Autodesk Inventor part; units mm, degrees
(part 2 of 2)
  line L680 (-7.1521, 71.8798) -> (-10.036, 76.875)
  line L681 (-4.554, 73.3798) -> (-7.4379, 78.375)
  line L682 (4.0979, 78.375) -> (1.214, 83.3701)
  line L683 (1.214, 83.3701) -> (-1.67, 83.3701)
  line L684 (-4.554, 83.3701) -> (-1.67, 83.3701)
  line L685 (-10.036, 76.875) -> (-15.804, 76.875)
  line L686 (-10.036, 79.875) -> (-15.804, 79.875)
  line L687 (-7.4379, 78.375) -> (-4.554, 83.3701)
  line L688 (-7.1521, 84.8701) -> (-10.036, 79.875)
  line L689 (3.8121, 84.8701) -> (6.696, 79.875)
  line L690 (60.0621, 65.3846) -> (62.946, 70.3798)
  line L691 (57.464, 66.8846) -> (60.3479, 71.8798)
  line L692 (62.946, 60.3894) -> (60.0621, 65.3846)
  line L693 (57.464, 63.8846) -> (60.3479, 58.8894)
  line L694 (51.696, 63.8846) -> (57.464, 63.8846)
  line L695 (51.696, 66.8846) -> (57.464, 66.8846)
  line L696 (51.696, 76.875) -> (57.464, 76.875)
  line L697 (51.696, 79.875) -> (57.464, 79.875)
  line L698 (57.464, 76.875) -> (60.3479, 71.8798)
  line L699 (60.0621, 78.375) -> (62.946, 73.3798)
  line L700 (62.946, 83.3701) -> (60.0621, 78.375)
  line L701 (57.464, 79.875) -> (60.3479, 84.8701)
  line L702 (23.714, 73.3798) -> (20.83, 73.3798)
  line L703 (29.196, 76.875) -> (26.3121, 71.8798)
  line L704 (26.5979, 78.375) -> (23.714, 73.3798)
  line L705 (34.964, 76.875) -> (29.196, 76.875)
  line L706 (20.83, 83.3701) -> (23.714, 83.3701)
  line L707 (23.714, 83.3701) -> (26.5979, 78.375)
  line L708 (34.964, 79.875) -> (29.196, 79.875)
  line L709 (29.196, 79.875) -> (26.3121, 84.8701)
  line L710 (37.8479, 84.8701) -> (34.964, 79.875)
  line L711 (37.8479, 71.8798) -> (34.964, 76.875)
  line L712 (6.696, 63.8846) -> (12.464, 63.8846)
  line L713 (6.696, 66.8846) -> (12.464, 66.8846)
  line L714 (6.696, 76.875) -> (12.464, 76.875)
  line L715 (6.696, 79.875) -> (12.464, 79.875)
  line L716 (12.464, 79.875) -> (15.3479, 84.8701)
  line L717 (12.464, 76.875) -> (15.3479, 71.8798)
  line L718 (17.946, 83.3701) -> (15.0621, 78.375)
  line L719 (20.83, 83.3701) -> (17.946, 83.3701)
  line L720 (15.0621, 78.375) -> (17.946, 73.3798)
  line L721 (17.946, 73.3798) -> (20.83, 73.3798)
  line L722 (-29.9379, 78.375) -> (-27.054, 83.3701)
  line L723 (-33.4021, 78.375) -> (-29.6521, 84.8701)
  line L724 (-27.054, 83.3701) -> (-21.286, 83.3701)
  line L725 (-21.286, 83.3701) -> (-18.4021, 78.375)
  line L726 (-15.804, 79.875) -> (-18.6879, 84.8701)
  line L727 (48.8121, 71.8798) -> (51.696, 76.875)
  line L728 (43.33, 73.3798) -> (40.446, 73.3798)
  line L729 (46.214, 73.3798) -> (49.0979, 78.375)
  line L730 (40.446, 73.3798) -> (37.5621, 78.375)
  line L731 (43.33, 73.3798) -> (46.214, 73.3798)
  line L732 (51.696, 11.923) -> (57.464, 11.923)
  line L733 (62.946, 8.4279) -> (60.0621, 13.423)
  line L734 (57.464, 11.923) -> (60.3479, 6.9279)
  line L735 (4.0979, 52.3942) -> (1.214, 57.3894)
  line L736 (-1.67, 47.399) -> (1.214, 47.399)
  line L737 (1.214, 57.3894) -> (-1.67, 57.3894)
  line L738 (-1.67, 47.399) -> (-4.554, 47.399)
  line L739 (-4.554, 57.3894) -> (-1.67, 57.3894)
  line L740 (-4.554, 47.399) -> (-7.4379, 52.3942)
  line L741 (-7.1521, 45.899) -> (-10.036, 50.8942)
  line L742 (-7.4379, 52.3942) -> (-4.554, 57.3894)
  line L743 (-7.1521, 58.8894) -> (-10.036, 53.8942)
  line L744 (1.214, 47.399) -> (4.0979, 52.3942)
  line L745 (-7.1521, 19.9182) -> (-10.036, 14.923)
  line L746 (-7.1521, 6.9279) -> (-10.036, 11.923)
  line L747 (-1.67, 18.4182) -> (-4.554, 18.4182)
  line L748 (-1.67, 18.4182) -> (1.214, 18.4182)
  line L749 (-4.554, 18.4182) -> (-7.4379, 13.423)
  line L750 (-7.4379, 13.423) -> (-4.554, 8.4279)
  line L751 (-4.554, 8.4279) -> (-1.67, 8.4279)
  line L752 (1.214, 8.4279) -> (-1.67, 8.4279)
  line L753 (4.0979, 13.423) -> (1.214, 8.4279)
  line L754 (3.8121, 6.9279) -> (6.696, 11.923)
  line L755 (26.5979, 13.423) -> (23.714, 18.4182)
  line L756 (23.714, 8.4279) -> (26.5979, 13.423)
  line L757 (20.83, 8.4279) -> (23.714, 8.4279)
  line L758 (23.714, 18.4182) -> (20.83, 18.4182)
  line L759 (20.83, 8.4279) -> (17.946, 8.4279)
  line L760 (17.946, 18.4182) -> (20.83, 18.4182)
  line L761 (17.946, 8.4279) -> (15.0621, 13.423)
  line L762 (12.464, 11.923) -> (15.3479, 6.9279)
  line L763 (15.0621, 13.423) -> (17.946, 18.4182)
  line L764 (12.464, 14.923) -> (15.3479, 19.9182)
  line L765 (29.196, 14.923) -> (26.3121, 19.9182)
  line L766 (29.196, 11.923) -> (26.3121, 6.9279)
  line L767 (34.964, 14.923) -> (29.196, 14.923)
  line L768 (34.964, 11.923) -> (29.196, 11.923)
  line L769 (43.33, 21.4182) -> (40.446, 21.4182)
  line L770 (43.33, 21.4182) -> (46.214, 21.4182)
  line L771 (43.33, 18.4182) -> (40.446, 18.4182)
  line L772 (43.33, 18.4182) -> (46.214, 18.4182)
  line L773 (37.8479, 19.9182) -> (34.964, 14.923)
  line L774 (40.446, 18.4182) -> (37.5621, 13.423)
  line L775 (48.8121, 19.9182) -> (51.696, 14.923)
  line L776 (46.214, 18.4182) -> (49.0979, 13.423)
  line L777 (37.8479, 6.9279) -> (34.964, 11.923)
  line L778 (37.5621, 13.423) -> (40.446, 8.4279)
  line L779 (40.446, 8.4279) -> (43.33, 8.4279)
  line L780 (46.214, 8.4279) -> (43.33, 8.4279)
  line L781 (49.0979, 13.423) -> (46.214, 8.4279)
  line L782 (48.8121, 6.9279) -> (51.696, 11.923)
  line L783 (-18.4021, 26.4134) -> (-21.286, 21.4182)
  line L784 (-15.804, 24.9134) -> (-18.6879, 19.9182)
  line L785 (-18.4021, 13.423) -> (-21.286, 18.4182)
  line L786 (-21.286, 8.4279) -> (-18.4021, 13.423)
  line L787 (-15.804, 11.923) -> (-18.6879, 6.9279)
  line L788 (-10.036, 11.923) -> (-15.804, 11.923)
  line L789 (-10.036, 14.923) -> (-15.804, 14.923)
  line L790 (-15.804, 14.923) -> (-18.6879, 19.9182)
  line L791 (-27.054, 8.4279) -> (-21.286, 8.4279)
  line L792 (-21.286, 21.4182) -> (-27.054, 21.4182)
  line L793 (-21.286, 18.4182) -> (-27.054, 18.4182)
  line L794 (-29.9379, 13.423) -> (-27.054, 8.4279)
  line L795 (-27.054, 18.4182) -> (-29.9379, 13.423)
  line L796 (-27.054, 21.4182) -> (-29.9379, 26.4134)
  line L797 (-32.969, 14.173) -> (-29.6521, 19.9182)
  line L798 (-29.6521, 19.9182) -> (-33.4021, 26.4134)
  line L799 (46.214, 21.4182) -> (49.0979, 26.4134)
  line L800 (37.8479, 19.9182) -> (34.964, 24.9134)
  line L801 (40.446, 21.4182) -> (37.5621, 26.4134)
  line L802 (37.5621, 26.4134) -> (40.446, 31.4086)
  line L803 (37.8479, 32.9086) -> (34.964, 27.9134)
  line L804 (-1.67, 21.4182) -> (1.214, 21.4182)
  line L805 (-1.67, 21.4182) -> (-4.554, 21.4182)
  line L806 (-7.1521, 19.9182) -> (-10.036, 24.9134)
  line L807 (-4.554, 21.4182) -> (-7.4379, 26.4134)
  line L808 (1.214, 31.4086) -> (-1.67, 31.4086)
  line L809 (-7.4379, 26.4134) -> (-4.554, 31.4086)
  line L810 (-7.1521, 32.9086) -> (-10.036, 27.9134)
  line L811 (23.714, 21.4182) -> (20.83, 21.4182)
  line L812 (17.946, 21.4182) -> (20.83, 21.4182)
  line L813 (29.196, 24.9134) -> (26.3121, 19.9182)
  line L814 (12.464, 24.9134) -> (15.3479, 19.9182)
  line L815 (15.0621, 26.4134) -> (17.946, 21.4182)
  line L816 (26.5979, 26.4134) -> (23.714, 21.4182)
  line L817 (34.964, 24.9134) -> (29.196, 24.9134)
  line L818 (34.964, 27.9134) -> (29.196, 27.9134)
  line L819 (20.83, 31.4086) -> (23.714, 31.4086)
  line L820 (23.714, 31.4086) -> (26.5979, 26.4134)
  line L821 (29.196, 27.9134) -> (26.3121, 32.9086)
  line L822 (1.214, 18.4182) -> (4.0979, 13.423)
  line L823 (3.8121, 19.9182) -> (6.696, 14.923)
  line L824 (6.696, 11.923) -> (12.464, 11.923)
  line L825 (6.696, 14.923) -> (12.464, 14.923)
  line L826 (1.214, 21.4182) -> (4.0979, 26.4134)
  line L827 (3.8121, 19.9182) -> (6.696, 24.9134)
  line L828 (4.0979, 26.4134) -> (1.214, 31.4086)
  line L829 (3.8121, 32.9086) -> (6.696, 27.9134)
  line L830 (6.696, 24.9134) -> (12.464, 24.9134)
  line L831 (6.696, 27.9134) -> (12.464, 27.9134)
  line L832 (12.464, 27.9134) -> (15.3479, 32.9086)
  line L833 (17.946, 31.4086) -> (15.0621, 26.4134)
  line L834 (57.464, 37.9038) -> (60.3479, 32.9086)
  line L835 (62.946, 34.4086) -> (60.0621, 39.4038)
  line L836 (51.696, 37.9038) -> (57.464, 37.9038)
  line L837 (51.696, 40.9038) -> (57.464, 40.9038)
  line L838 (60.0621, 39.4038) -> (62.946, 44.399)
  line L839 (57.464, 40.9038) -> (60.3479, 45.899)
  line L840 (46.214, 31.4086) -> (43.33, 31.4086)
  line L841 (40.446, 31.4086) -> (43.33, 31.4086)
  line L842 (48.8121, 32.9086) -> (51.696, 37.9038)
  line L843 (46.214, 34.4086) -> (43.33, 34.4086)
  line L844 (49.0979, 39.4038) -> (46.214, 34.4086)
  line L845 (40.446, 34.4086) -> (43.33, 34.4086)
  line L846 (48.8121, 45.899) -> (51.696, 40.9038)
  line L847 (46.214, 44.399) -> (49.0979, 39.4038)
  line L848 (43.33, 44.399) -> (46.214, 44.399)
  line L849 (43.33, 44.399) -> (40.446, 44.399)
  line L850 (20.83, 34.4086) -> (23.714, 34.4086)
  line L851 (29.196, 37.9038) -> (26.3121, 32.9086)
  line L852 (34.964, 37.9038) -> (29.196, 37.9038)
  line L853 (37.8479, 32.9086) -> (34.964, 37.9038)
  line L854 (23.714, 34.4086) -> (26.5979, 39.4038)
  line L855 (34.964, 40.9038) -> (29.196, 40.9038)
  line L856 (37.5621, 39.4038) -> (40.446, 34.4086)
  line L857 (23.714, 44.399) -> (20.83, 44.399)
  line L858 (26.5979, 39.4038) -> (23.714, 44.399)
  line L859 (29.196, 40.9038) -> (26.3121, 45.899)
  line L860 (40.446, 44.399) -> (37.5621, 39.4038)
  line L861 (37.8479, 45.899) -> (34.964, 40.9038)
  line L862 (3.8121, 45.899) -> (6.696, 40.9038)
  line L863 (1.214, 44.399) -> (4.0979, 39.4038)
  line L864 (6.696, 40.9038) -> (12.464, 40.9038)
  line L865 (6.696, 37.9038) -> (12.464, 37.9038)
  line L866 (4.0979, 39.4038) -> (1.214, 34.4086)
  line L867 (3.8121, 32.9086) -> (6.696, 37.9038)
  line L868 (-15.804, 27.9134) -> (-18.6879, 32.9086)
  line L869 (-10.036, 27.9134) -> (-15.804, 27.9134)
  line L870 (-10.036, 24.9134) -> (-15.804, 24.9134)
  line L871 (-4.554, 31.4086) -> (-1.67, 31.4086)
  line L872 (-15.804, 40.9038) -> (-18.6879, 45.899)
  line L873 (-10.036, 40.9038) -> (-15.804, 40.9038)
  line L874 (-15.804, 37.9038) -> (-18.6879, 32.9086)
  line L875 (-10.036, 37.9038) -> (-15.804, 37.9038)
  line L876 (-7.1521, 45.899) -> (-10.036, 40.9038)
  line L877 (-1.67, 44.399) -> (-4.554, 44.399)
  line L878 (-4.554, 44.399) -> (-7.4379, 39.4038)
  line L879 (-7.1521, 32.9086) -> (-10.036, 37.9038)
  line L880 (-1.67, 44.399) -> (1.214, 44.399)
  line L881 (-7.4379, 39.4038) -> (-4.554, 34.4086)
  line L882 (-4.554, 34.4086) -> (-1.67, 34.4086)
  line L883 (1.214, 34.4086) -> (-1.67, 34.4086)
  line L884 (20.83, 31.4086) -> (17.946, 31.4086)
  line L885 (12.464, 37.9038) -> (15.3479, 32.9086)
  line L886 (20.83, 34.4086) -> (17.946, 34.4086)
  line L887 (17.946, 34.4086) -> (15.0621, 39.4038)
  line L888 (15.0621, 39.4038) -> (17.946, 44.399)
  line L889 (17.946, 44.399) -> (20.83, 44.399)
  line L890 (17.946, 47.399) -> (20.83, 47.399)
  line L891 (12.464, 40.9038) -> (15.3479, 45.899)
  line L892 (48.8121, 45.899) -> (51.696, 50.8942)
  line L893 (51.696, 50.8942) -> (57.464, 50.8942)
  line L894 (51.696, 53.8942) -> (57.464, 53.8942)
  line L895 (57.464, 50.8942) -> (60.3479, 45.899)
  line L896 (60.0621, 52.3942) -> (62.946, 47.399)
  line L897 (62.946, 57.3894) -> (60.0621, 52.3942)
  line L898 (57.464, 53.8942) -> (60.3479, 58.8894)
  line L899 (48.8121, 58.8894) -> (51.696, 53.8942)
  line L900 (29.196, 53.8942) -> (26.3121, 58.8894)
  line L901 (29.196, 50.8942) -> (26.3121, 45.899)
  line L902 (34.964, 50.8942) -> (29.196, 50.8942)
  line L903 (34.964, 53.8942) -> (29.196, 53.8942)
  line L904 (37.8479, 45.899) -> (34.964, 50.8942)
  line L905 (37.8479, 58.8894) -> (34.964, 53.8942)
  line L906 (49.0979, 52.3942) -> (46.214, 57.3894)
  line L907 (46.214, 47.399) -> (49.0979, 52.3942)
  line L908 (46.214, 57.3894) -> (43.33, 57.3894)
  line L909 (40.446, 57.3894) -> (43.33, 57.3894)
  line L910 (43.33, 47.399) -> (40.446, 47.399)
  line L911 (37.5621, 52.3942) -> (40.446, 57.3894)
  line L912 (40.446, 47.399) -> (37.5621, 52.3942)
  line L913 (43.33, 47.399) -> (46.214, 47.399)
  line L914 (20.83, 57.3894) -> (17.946, 57.3894)
  line L915 (20.83, 57.3894) -> (23.714, 57.3894)
  line L916 (23.714, 57.3894) -> (26.5979, 52.3942)
  line L917 (12.464, 53.8942) -> (15.3479, 58.8894)
  line L918 (17.946, 57.3894) -> (15.0621, 52.3942)
  line L919 (6.696, 53.8942) -> (12.464, 53.8942)
  line L920 (3.8121, 58.8894) -> (6.696, 53.8942)
  line L921 (26.5979, 52.3942) -> (23.714, 47.399)
  line L922 (23.714, 47.399) -> (20.83, 47.399)
  line L923 (6.696, 50.8942) -> (12.464, 50.8942)
  line L924 (15.0621, 52.3942) -> (17.946, 47.399)
  line L925 (12.464, 50.8942) -> (15.3479, 45.899)
  line L926 (3.8121, 45.899) -> (6.696, 50.8942)
  line L927 (-18.4021, 52.3942) -> (-21.286, 47.399)
  line L928 (-32.969, 51.6442) -> (-29.6521, 45.899)
  line L929 (-27.054, 47.399) -> (-29.9379, 52.3942)
  line L930 (-21.286, 47.399) -> (-27.054, 47.399)
  line L931 (-15.804, 50.8942) -> (-18.6879, 45.899)
  line L932 (-10.036, 50.8942) -> (-15.804, 50.8942)
  line L933 (-10.036, 53.8942) -> (-15.804, 53.8942)
  line L934 (-21.286, 57.3894) -> (-18.4021, 52.3942)
  line L935 (-27.054, 57.3894) -> (-21.286, 57.3894)
  line L936 (-29.9379, 52.3942) -> (-27.054, 57.3894)
  line L937 (-15.804, 53.8942) -> (-18.6879, 58.8894)
  line L938 (49.0979, 26.4134) -> (46.214, 31.4086)
  line L939 (48.8121, 32.9086) -> (51.696, 27.9134)
  line L940 (51.696, 27.9134) -> (57.464, 27.9134)
  line L941 (48.8121, 19.9182) -> (51.696, 24.9134)
  line L942 (57.464, 27.9134) -> (60.3479, 32.9086)
  line L943 (51.696, 24.9134) -> (57.464, 24.9134)
  line L944 (62.946, 31.4086) -> (60.0621, 26.4134)
  line L945 (57.464, 24.9134) -> (60.3479, 19.9182)
  line L946 (51.696, 14.923) -> (57.464, 14.923)
  line L947 (57.464, 14.923) -> (60.3479, 19.9182)
  line L948 (60.0621, 13.423) -> (62.946, 18.4182)
  line L949 (60.0621, 26.4134) -> (62.946, 21.4182)
  line L950 (-21.286, 31.4086) -> (-18.4021, 26.4134)
  line L951 (-29.9379, 26.4134) -> (-27.054, 31.4086)
  line L952 (-33.4021, 26.4134) -> (-29.6521, 32.9086)
  line L953 (-27.054, 31.4086) -> (-21.286, 31.4086)
  line L954 (-27.054, 34.4086) -> (-21.286, 34.4086)
  line L955 (-33.4021, 39.4038) -> (-29.6521, 32.9086)
  line L956 (-29.9379, 39.4038) -> (-27.054, 34.4086)
  line L957 (-21.286, 34.4086) -> (-18.4021, 39.4038)
  line L958 (-18.4021, 39.4038) -> (-21.286, 44.399)
  line L959 (-21.286, 44.399) -> (-27.054, 44.399)
  line L960 (-27.054, 44.399) -> (-29.9379, 39.4038)
  line L961 (-29.6521, 45.899) -> (-33.4021, 39.4038)
  line L962 (-32.969, -39.2885) -> (-29.6521, -45.0337)
  line L963 (-29.6521, -45.0337) -> (-32.969, -50.7789)
  line L964 (-29.6521, 6.9279) -> (-32.969, 1.1827)
  line L965 (-29.6521, 6.9279) -> (-32.969, 12.673)
  line L966 (-32.969, 64.6346) -> (-29.6521, 58.8894)
  line L967 (-29.6521, 58.8894) -> (-32.969, 53.1442)
  line L968 (-32.969, 64.6346) -> (-33.4021, 65.3846)
  line L969 (-32.969, 66.1346) -> (-33.4021, 65.3846)
  line L970 (-32.969, 51.6442) -> (-33.4021, 52.3942)
  line L971 (-32.969, 53.1442) -> (-33.4021, 52.3942)
  line L972 (37.8479, 136.8317) -> (34.964, 141.8269)
  line L973 (37.5621, 143.3269) -> (40.446, 138.3317)
  line L974 (40.446, 138.3317) -> (43.33, 138.3317)
  line L975 (46.214, 138.3317) -> (43.33, 138.3317)
  line L976 (20.83, 135.3317) -> (17.946, 135.3317)
  line L977 (17.946, 138.3317) -> (15.0621, 143.3269)
  line L978 (20.83, 138.3317) -> (17.946, 138.3317)
  line L979 (20.83, 138.3317) -> (23.714, 138.3317)
  line L980 (23.714, 138.3317) -> (26.5979, 143.3269)
  line L981 (29.196, 141.8269) -> (26.3121, 136.8317)
  line L982 (6.696, 128.8365) -> (12.464, 128.8365)
  line L983 (6.696, 131.8365) -> (12.464, 131.8365)
  line L984 (17.946, 135.3317) -> (15.0621, 130.3365)
  line L985 (12.464, 131.8365) -> (15.3479, 136.8317)
  line L986 (6.696, 141.8269) -> (12.464, 141.8269)
  line L987 (12.464, 141.8269) -> (15.3479, 136.8317)
  line L988 (3.8121, 136.8317) -> (6.696, 141.8269)
  line L989 (4.0979, 143.3269) -> (1.214, 138.3317)
  line L990 (34.964, 141.8269) -> (29.196, 141.8269)
  line L991 (-7.4379, 117.3461) -> (-4.554, 112.3509)
  line L992 (-10.036, 118.8461) -> (-15.804, 118.8461)
  line L993 (-10.036, 115.8461) -> (-15.804, 115.8461)
  line L994 (-15.804, 115.8461) -> (-18.6879, 110.8509)
  line L995 (-21.286, 112.3509) -> (-18.4021, 117.3461)
  line L996 (-1.67, 125.3413) -> (-4.554, 125.3413)
  line L997 (3.8121, 123.8413) -> (6.696, 128.8365)
  line L998 (1.214, 125.3413) -> (4.0979, 130.3365)
  line L999 (-4.554, 125.3413) -> (-7.4379, 130.3365)
  line L1000 (-7.1521, 123.8413) -> (-10.036, 128.8365)
  line L1001 (4.0979, 130.3365) -> (1.214, 135.3317)
  line L1002 (3.8121, 136.8317) -> (6.696, 131.8365)
  line L1003 (1.214, 135.3317) -> (-1.67, 135.3317)
  line L1004 (-4.554, 135.3317) -> (-1.67, 135.3317)
  line L1005 (1.214, 138.3317) -> (-1.67, 138.3317)
  line L1006 (-7.4379, 130.3365) -> (-4.554, 135.3317)
  line L1007 (-4.554, 138.3317) -> (-1.67, 138.3317)
  line L1008 (-15.804, 118.8461) -> (-18.6879, 123.8413)
  line L1009 (-18.4021, 117.3461) -> (-21.286, 122.3413)
  line L1010 (-27.054, 112.3509) -> (-21.286, 112.3509)
  line L1011 (-29.9379, 117.3461) -> (-27.054, 112.3509)
  line L1012 (-21.286, 122.3413) -> (-27.054, 122.3413)
  line L1013 (-18.4021, 130.3365) -> (-21.286, 125.3413)
  line L1014 (-21.286, 125.3413) -> (-27.054, 125.3413)
  line L1015 (-27.054, 122.3413) -> (-29.9379, 117.3461)
  line L1016 (-32.969, 118.0961) -> (-29.6521, 123.8413)
  line L1017 (-29.6521, 123.8413) -> (-33.4021, 130.3365)
  line L1018 (-27.054, 125.3413) -> (-29.9379, 130.3365)
  line L1019 (-4.554, 112.3509) -> (-1.67, 112.3509)
  line L1020 (-7.1521, 110.8509) -> (-10.036, 115.8461)
  line L1021 (-4.554, 122.3413) -> (-7.4379, 117.3461)
  line L1022 (-1.67, 122.3413) -> (-4.554, 122.3413)
  line L1023 (4.0979, 117.3461) -> (1.214, 112.3509)
  line L1024 (-7.1521, 123.8413) -> (-10.036, 118.8461)
  line L1025 (-1.67, 122.3413) -> (1.214, 122.3413)
  line L1026 (-1.67, 125.3413) -> (1.214, 125.3413)
  line L1027 (1.214, 122.3413) -> (4.0979, 117.3461)
  line L1028 (3.8121, 123.8413) -> (6.696, 118.8461)
  line L1029 (3.8121, 110.8509) -> (6.696, 115.8461)
  line L1030 (6.696, 118.8461) -> (12.464, 118.8461)
  line L1031 (6.696, 115.8461) -> (12.464, 115.8461)
  line L1032 (1.214, 112.3509) -> (-1.67, 112.3509)
  line L1033 (-15.804, 131.8365) -> (-18.6879, 136.8317)
  line L1034 (-10.036, 131.8365) -> (-15.804, 131.8365)
  line L1035 (-10.036, 128.8365) -> (-15.804, 128.8365)
  line L1036 (-7.1521, 136.8317) -> (-10.036, 131.8365)
  line L1037 (-15.804, 128.8365) -> (-18.6879, 123.8413)
  line L1038 (-7.4379, 143.3269) -> (-4.554, 138.3317)
  line L1039 (-7.1521, 136.8317) -> (-10.036, 141.8269)
  line L1040 (-10.036, 141.8269) -> (-15.804, 141.8269)
  line L1041 (-15.804, 141.8269) -> (-18.6879, 136.8317)
  line L1042 (-29.9379, 130.3365) -> (-27.054, 135.3317)
  line L1043 (-21.286, 135.3317) -> (-18.4021, 130.3365)
  line L1044 (-33.4021, 130.3365) -> (-29.6521, 136.8317)
  line L1045 (-27.054, 135.3317) -> (-21.286, 135.3317)
  line L1046 (-27.054, 138.3317) -> (-21.286, 138.3317)
  line L1047 (-33.4021, 143.3269) -> (-29.6521, 136.8317)
  line L1048 (-29.9379, 143.3269) -> (-27.054, 138.3317)
  line L1049 (-21.286, 138.3317) -> (-18.4021, 143.3269)
  line L1050 (57.464, 118.8461) -> (60.3479, 123.8413)
  line L1051 (60.0621, 117.3461) -> (62.946, 122.3413)
  line L1052 (51.696, 118.8461) -> (57.464, 118.8461)
  line L1053 (51.696, 115.8461) -> (57.464, 115.8461)
  line L1054 (57.464, 115.8461) -> (60.3479, 110.8509)
  line L1055 (62.946, 112.3509) -> (60.0621, 117.3461)
  line L1056 (12.464, 115.8461) -> (15.3479, 110.8509)
  line L1057 (17.946, 112.3509) -> (15.0621, 117.3461)
  line L1058 (12.464, 118.8461) -> (15.3479, 123.8413)
  line L1059 (15.0621, 117.3461) -> (17.946, 122.3413)
  line L1060 (17.946, 122.3413) -> (20.83, 122.3413)
  line L1061 (20.83, 112.3509) -> (17.946, 112.3509)
  line L1062 (23.714, 122.3413) -> (20.83, 122.3413)
  line L1063 (29.196, 118.8461) -> (26.3121, 123.8413)
  line L1064 (26.5979, 117.3461) -> (23.714, 122.3413)
  line L1065 (34.964, 118.8461) -> (29.196, 118.8461)
  line L1066 (34.964, 115.8461) -> (29.196, 115.8461)
  line L1067 (20.83, 112.3509) -> (23.714, 112.3509)
  line L1068 (23.714, 112.3509) -> (26.5979, 117.3461)
  line L1069 (29.196, 115.8461) -> (26.3121, 110.8509)
  line L1070 (37.8479, 110.8509) -> (34.964, 115.8461)
  line L1071 (37.8479, 123.8413) -> (34.964, 118.8461)
  line L1072 (40.446, 122.3413) -> (37.5621, 117.3461)
  line L1073 (43.33, 122.3413) -> (40.446, 122.3413)
  line L1074 (43.33, 122.3413) -> (46.214, 122.3413)
  line L1075 (48.8121, 123.8413) -> (51.696, 118.8461)
  line L1076 (46.214, 122.3413) -> (49.0979, 117.3461)
  line L1077 (37.5621, 117.3461) -> (40.446, 112.3509)
  line L1078 (40.446, 112.3509) -> (43.33, 112.3509)
  line L1079 (46.214, 112.3509) -> (43.33, 112.3509)
  line L1080 (49.0979, 117.3461) -> (46.214, 112.3509)
  line L1081 (48.8121, 110.8509) -> (51.696, 115.8461)
  line L1082 (23.714, 125.3413) -> (20.83, 125.3413)
  line L1083 (17.946, 125.3413) -> (20.83, 125.3413)
  line L1084 (12.464, 128.8365) -> (15.3479, 123.8413)
  line L1085 (15.0621, 130.3365) -> (17.946, 125.3413)
  line L1086 (26.5979, 130.3365) -> (23.714, 125.3413)
  line L1087 (34.964, 128.8365) -> (29.196, 128.8365)
  line L1088 (34.964, 131.8365) -> (29.196, 131.8365)
  line L1089 (20.83, 135.3317) -> (23.714, 135.3317)
  line L1090 (23.714, 135.3317) -> (26.5979, 130.3365)
  line L1091 (29.196, 131.8365) -> (26.3121, 136.8317)
  line L1092 (29.196, 128.8365) -> (26.3121, 123.8413)
  line L1093 (57.464, 128.8365) -> (60.3479, 123.8413)
  line L1094 (60.0621, 130.3365) -> (62.946, 125.3413)
  line L1095 (51.696, 128.8365) -> (57.464, 128.8365)
  line L1096 (48.8121, 123.8413) -> (51.696, 128.8365)
  line L1097 (62.946, 135.3317) -> (60.0621, 130.3365)
  line L1098 (51.696, 131.8365) -> (57.464, 131.8365)
  line L1099 (57.464, 131.8365) -> (60.3479, 136.8317)
  line L1100 (48.8121, 136.8317) -> (51.696, 131.8365)
  line L1101 (49.0979, 130.3365) -> (46.214, 135.3317)
  line L1102 (46.214, 125.3413) -> (49.0979, 130.3365)
  line L1103 (43.33, 125.3413) -> (46.214, 125.3413)
  line L1104 (43.33, 125.3413) -> (40.446, 125.3413)
  line L1105 (37.8479, 123.8413) -> (34.964, 128.8365)
  line L1106 (40.446, 125.3413) -> (37.5621, 130.3365)
  line L1107 (46.214, 135.3317) -> (43.33, 135.3317)
  line L1108 (40.446, 135.3317) -> (43.33, 135.3317)
  line L1109 (37.5621, 130.3365) -> (40.446, 135.3317)
  line L1110 (37.8479, 136.8317) -> (34.964, 131.8365)
  line L1111 (57.464, 141.8269) -> (60.3479, 136.8317)
  line L1112 (48.8121, 136.8317) -> (51.696, 141.8269)
  line L1113 (49.0979, 143.3269) -> (46.214, 138.3317)
  line L1114 (62.946, 138.3317) -> (60.0621, 143.3269)
  line L1115 (51.696, 141.8269) -> (57.464, 141.8269)
  line L1116 (-32.969, 116.5961) -> (-29.6521, 110.8509)
  line L1117 (-29.6521, 110.8509) -> (-32.969, 105.1057)
  line L1118 (-32.969, 103.6057) -> (-33.4021, 104.3557)
  line L1119 (-32.969, 105.1057) -> (-33.4021, 104.3557)
  line L1120 (-32.969, 116.5961) -> (-33.4021, 117.3461)
  line L1121 (-32.969, 118.0961) -> (-33.4021, 117.3461)
  line L1122 (-32.969, -52.2789) -> (-33.4021, -51.5289)
  line L1123 (-32.969, -50.7789) -> (-33.4021, -51.5289)
  line L1124 (-32.969, -37.7885) -> (-33.4021, -38.5385)
  line L1125 (-32.969, -39.2885) -> (-33.4021, -38.5385)
  line L1126 (-32.969, 12.673) -> (-33.4021, 13.423)
  line L1127 (-32.9501, 14.2058) -> (-33.4021, 13.423)
  line L1128 (-7.1521, -96.9952) -> (-10.036, -101.9904)
  line L1129 (-10.036, -101.9904) -> (-15.804, -101.9904)
  line L1130 (-15.804, -101.9904) -> (-18.6879, -96.9952)
  line L1131 (3.8121, -96.9952) -> (6.696, -101.9904)
  line L1132 (6.696, -101.9904) -> (12.464, -101.9904)
  line L1133 (12.464, -101.9904) -> (15.3479, -96.9952)
  line L1134 (57.464, -101.9904) -> (60.3479, -96.9952)
  line L1135 (51.696, -101.9904) -> (57.464, -101.9904)
  line L1136 (37.8479, -96.9952) -> (34.964, -101.9904)
  line L1137 (34.964, -101.9904) -> (29.196, -101.9904)
  line L1138 (29.196, -101.9904) -> (26.3121, -96.9952)
  line L1139 (48.8121, -96.9952) -> (51.696, -101.9904)
  point P0 (0, 0)
  point P1 (14.5, 82.5)
  point P2 (14.5, -38)
  point P3 (3.676, -78)
  point P4 (12.6121, -98)
  point P5 (53.17, -77.5096)
  point P6 (-24.17, -51.5289)
  point P7 (-24.17, -51.5289)
  point P8 (60.67, -51.5289)
  point P9 (53.17, -51.5289)
  point P10 (-24.17, -51.5289)
  point P11 (53.17, -64.5192)
  point P12 (-24.17, 0.4327)
  point P13 (-24.17, 0.4327)
  point P14 (60.67, 0.4327)
  point P15 (53.17, 0.4327)
  point P16 (-24.17, 0.4327)
  point P17 (53.17, -12.5577)
  point P18 (-24.17, -38.5385)
  point P19 (-24.17, -38.5385)
  point P20 (53.17, -38.5385)
  point P21 (60.67, -38.5385)
  point P22 (53.17, -25.5481)
  point P23 (-24.17, -38.5385)
  point P24 (0, 13.8557)
  point P25 (14.5, 51.8557)
  point P26 (-24.17, 104.3557)
  point P27 (-24.17, 104.3557)
  point P28 (14.5, 27.1709)
  point P29 (60.67, 104.3557)
  point P30 (53.17, 104.3557)
  point P31 (-24.17, 104.3557)
  point P32 (53.17, 91.3653)
  point P33 (-24.17, 65.3846)
  point P34 (-24.17, 65.3846)
  point P35 (53.17, 65.3846)
  point P36 (60.67, 65.3846)
  point P37 (53.17, 78.375)
  point P38 (-24.17, 65.3846)
  point P39 (60.67, 13.423)
  point P40 (53.17, 13.423)
  point P41 (-24.17, 13.423)
  point P42 (-24.17, 13.423)
  point P43 (53.17, 39.4038)
  point P44 (53.17, 52.3942)
  point P45 (60.67, 52.3942)
  point P46 (-24.17, 52.3942)
  point P47 (-24.17, 52.3942)
  point P48 (53.17, 26.4134)
  point P49 (-24.17, 52.3942)
  point P50 (-24.17, 13.423)
  point P51 (14.5, 139.2018)
  point P52 (-24.17, 117.3461)
  point P53 (-24.17, 117.3461)
  point P54 (60.67, 117.3461)
  point P55 (53.17, 117.3461)
  point P56 (53.17, 130.3365)
  point P57 (53.17, 143.3269)
  point P58 (-24.17, 117.3461)
  point P59 (14.5, 5.4592)
  point P60 (14.5, 8.3965)
  point P61 (14.5, -7.5312)
  point P62 (14.5, -4.5938)
  point P63 (60.67, 131.3895)
  point P64 (60.67, 129.2835)
  point P65 (60.67, 116.2931)
  point P66 (60.67, 118.3991)
  point P67 (60.67, 105.4087)
  point P68 (60.67, 103.3027)
  point P69 (60.67, 90.3123)
  point P70 (60.67, 92.4183)
  point P71 (60.67, 77.322)
  point P72 (60.67, 79.428)
  point P73 (60.67, 66.4376)
  point P74 (60.67, 64.3316)
  point P75 (60.67, 53.4472)
  point P76 (60.67, 51.3412)
  point P77 (60.67, 40.4568)
  point P78 (60.67, 38.3508)
  point P79 (60.67, 27.4664)
  point P80 (60.67, 25.3604)
  point P81 (60.67, 14.476)
  point P82 (60.67, 12.37)
  point P83 (60.67, -0.6203)
  point P84 (60.67, 1.4857)
  point P85 (60.67, -11.5047)
  point P86 (60.67, -13.6107)
  point P87 (60.67, -26.6011)
  point P88 (60.67, -24.4951)
  point P89 (60.67, -39.5915)
  point P90 (60.67, -37.4855)
  point P91 (60.67, -50.4759)
  point P92 (60.67, -52.5819)
  point P93 (60.67, -65.5722)
  point P94 (60.67, -63.4662)
  point P95 (60.67, -76.4566)
  point P96 (60.67, -78.5626)
  point P97 (60.6098, -91.4487)
  point P98 (60.67, -89.447)
  point P99 (-31.67, -67.5192)
  point P100 (-31.67, -74.5096)
  point P101 (-31.67, -80.5096)
  point P102 (-31.67, -87.5)
  point P103 (-31.67, -54.5289)
  point P104 (-31.67, -61.5192)
  point P105 (-31.67, -48.5289)
  point P106 (-31.67, -41.5385)
  point P107 (-31.67, -28.5481)
  point P108 (-31.67, -35.5385)
  point P109 (-31.67, -22.5481)
  point P110 (-31.67, -15.5577)
  point P111 (-31.67, -9.5577)
  point P112 (-31.67, -2.5673)
  point P113 (-31.67, 10.423)
  point P114 (-31.67, 3.4327)
  point P115 (-31.67, 23.4134)
  point P116 (-31.67, 16.423)
  point P117 (-31.67, 36.4038)
  point P118 (-31.67, 29.4134)
  point P119 (-31.67, 42.4038)
  point P120 (-31.67, 49.3942)
  point P121 (-31.67, 55.3942)
  point P122 (-31.67, 62.3846)
  point P123 (-31.67, 68.3846)
  point P124 (-31.67, 75.375)
  point P125 (-31.67, 81.375)
  point P126 (-31.67, 88.3653)
  point P127 (-31.67, 94.3653)
  point P128 (-31.67, 101.3557)
  point P129 (-31.67, 107.3557)
  point P130 (-31.67, 114.3461)
  point P131 (-31.67, 120.3461)
  point P132 (-31.67, 127.3365)
  point P133 (-30.712, 138.6676)
  point P134 (-31.67, 133.3365)
  point P135 (58.1865, 140.5753)
  point P136 (56.2755, 141.8269)
  point P137 (48.6206, 142.5)
  point P138 (38.0394, 142.5)
  point P139 (26.1206, 142.5)
  point P140 (15.5394, 142.5)
  point P141 (3.6206, 142.5)
  point P142 (-6.9606, 142.5)
  point P143 (-18.8794, 142.5)
  point P144 (-28.6172, 141.0392)
  point P145 (49.3922, -98)
  point P146 (59.1847, -94.9804)
  point P147 (26.8922, -98)
  point P148 (37.2678, -98)
  point P149 (4.3922, -98)
  point P150 (14.7678, -98)
  point P151 (-18.1078, -98)
  point P152 (-7.7322, -98)
  dimension "d90" = 52.5
  dimension "d91" = 52.5
  dimension "d94" = 7.5
  dimension "d97" = 52.5
  dimension "d107" = 60
  dimension "d108" = 60
  dimension "d109" = 7.5
  dimension "d113" = 52.5
  constraints: 2216 end point, 19 coincident, 9 symmetric about line, 8 point on circle, 7 point on line, 4 centre point, 3 horizontal, 2 tangent, 1 horizontal alignment, 1 perpendicular, 1 vertical, 11 other
  measures "d90" horizontal distance of A7.centre point (14.5, 82.5)
  measures "d91" horizontal distance of A7.centre point (14.5, 82.5)
  measures "d94" radius of A28
  measures "d97" horizontal distance of point (14.5, -38) A0.centre
  measures "d107" distance from line of point (14.5, 82.5) L39
  measures "d108" distance from line of point (14.5, -38) L37
  measures "d109" distance from line of L32 A29.centre
  measures "d113" distance from line of A1.centre L34
extrude "Extrusion10" cut sketch "Sketch8" against normal up to surface (3 mm away) contours A28 L1047 L1044 L30 | L1017 L1016 L30 | A28 L33 L1049 L1046 L1048 | L1116 L1117 L30 | L614 L615 L30 | L39 L989 L1005 L1007 L1038 | L616 L723 L30 | L39 L980 L979 L978 L977 | L622 L623 L30 | L39 L38 L1113 L975 L974 L973 | L966 L967 L30 | L928 L961 L30 | A30 L1111 L1099 L1098 L1100 L1112 L1115 | L955 L952 L30 | L35 L1094 L1097 | L798 L797 L30 | L35 L1055 L1051 | L965 L964 L31 | L35 L533 L535 | L384 L385 L31 | L35 L611 L610 | L386 L493 L31 | L35 L699 L700 | L392 L393 L31 | L35 L692 L690 | L962 L963 L31 | L35 L896 L897 | L269 L270 L31 | L35 L835 L838 | L271 L156 L31 | L35 L949 L944 | L155 L154 L31 | L35 L36 L733 L948 | L36 L303 L305 | L1130 L53 L52 L51 L1128 L41 L32 | L36 L381 L380 | L1131 L65 L66 L67 L1133 L40 L41 | L36 L469 L470 | L36 L462 L460 | L1138 L91 L89 L84 L1136 L40 | L36 L188 L190 | L36 L266 L265 | L1139 L77 L78 L79 A31 L37 | L36 L129 L131 | L72 L73 L36 A31 | L34 L295 L293 L288 L754 L824 L762 | L34 L349 L350 L347 L292 L294 L298 | L47 L46 L45 L44 L43 L42 | L48 L49 L50 L106 L105 L104 | L68 L69 L70 L71 L57 L56 L55 L54 | L58 L96 L95 L93 L97 L59 L60 L61 | L118 L120 L124 L64 L63 L62 | L147 L134 L130 L76 L75 L74 | L80 L81 L82 L83 L92 L85 L87 L86 | L88 L90 L94 L145 L137 L138 | L98 L99 L100 L101 L102 L103 | L107 L108 L109 L217 L218 L220 | L110 L111 L112 L113 L122 L115 L117 L116 | L230 L237 L239 L121 L119 L114 | L127 L142 L144 L146 L128 L126 L125 L123 | L133 L148 L253 L242 L263 L132 | L135 L136 L143 L248 L250 L252 | L139 L140 L152 L151 L150 L149 L153 L141 | L157 L158 L159 L160 L161 L162 | L222 L219 L224 L165 L164 L163 | L166 L167 L168 L439 L440 L423 | L169 L170 L171 L172 L181 L174 L176 L175 | L428 L482 L411 L180 L178 L173 | L177 L179 L183 L234 L235 L232 | L186 L201 L203 L205 L187 L185 L184 L182 | L189 L264 L241 L254 L206 L193 | L192 L207 L421 L464 L463 L191 | L194 L195 L202 L398 L401 L403 | L197 L251 L249 L247 L204 L196 | L198 L199 L211 L210 L209 L208 L212 L200 | L214 L215 L268 L267 L216 L213 | L223 L225 L228 L231 L229 L227 L226 L221 | L233 L244 L246 L245 L243 L240 L238 L236 | L255 L256 L258 L261 L262 L260 L259 L257 | L272 L273 L274 L275 L276 L277 | L337 L334 L339 L280 L279 L278 | L281 L282 L283 L787 L788 L746 | L284 L285 L286 L287 L296 L289 L291 L290 | L301 L316 L318 L320 L302 L300 L299 L297 | L304 L379 L356 L369 L321 L308 | L307 L322 L782 L732 L734 L306 | L309 L310 L317 L766 L768 L777 | L312 L366 L364 L362 L319 L311 | L313 L314 L326 L325 L324 L323 L327 L315 | L329 L330 L383 L382 L331 L328 | L333 L335 L458 L456 L496 L332 | L338 L340 L343 L346 L344 L342 L341 L336 | L345 L352 L354 L486 L485 L459 | L348 L359 L361 L360 L358 L355 L353 L351 | L357 L378 L471 L467 L442 L368 | L365 L367 L480 L478 L479 L363 | L370 L371 L373 L376 L377 L375 L374 L372 | L455 L450 L422 L437 L438 L387 | L388 L389 L391 L492 L494 L495 | L436 L435 L434 L394 L395 L390 | L405 L406 L408 L409 L407 L404 L397 L396 | L399 L473 L475 L481 L402 L400 | L483 L433 L448 L484 L487 L410 | L412 L415 L420 L419 L418 L417 L416 L413 | L497 L466 L468 L461 L465 L414 | L430 L431 L429 L432 L427 L426 L425 L424 | L443 L499 L501 L498 L500 L444 L445 L441 | L447 L451 L457 L454 L453 L452 L449 L446 | L472 L491 L490 L488 L489 L476 L477 L474 | L502 L503 L504 L505 L506 L507 | L567 L564 L569 L510 L509 L508 | L511 L512 L513 L994 L993 L1020 | L514 L515 L516 L517 L526 L519 L521 L520 | L1029 L1031 L1056 L525 L523 L518 | L522 L524 L528 L579 L580 L577 | L531 L546 L548 L550 L532 L530 L529 L527 | L534 L609 L586 L599 L551 L538 | L537 L552 L1081 L1053 L1054 L536 | L539 L540 L547 L1069 L1066 L1070 | L542 L596 L594 L592 L549 L541 | L543 L544 L556 L555 L554 L553 L557 L545 | L559 L560 L613 L612 L561 L558 | L563 L565 L688 L686 L726 L562 | L568 L570 L573 L576 L574 L572 L571 L566 | L575 L582 L584 L716 L715 L689 | L578 L589 L591 L590 L588 L585 L583 L581 | L587 L608 L701 L697 L672 L598 | L595 L597 L710 L708 L709 L593 | L600 L601 L603 L606 L607 L605 L604 L602 | L685 L680 L652 L667 L668 L617 | L618 L619 L621 L722 L724 L725 | L666 L665 L664 L624 L625 L620 | L635 L636 L638 L639 L637 L634 L627 L626 | L631 L633 L905 L903 L900 L628 | L629 L703 L705 L711 L632 L630 | L713 L663 L678 L714 L717 L640 | L641 L917 L919 L920 L658 L712 | L642 L645 L650 L649 L648 L647 L646 L643 | L727 L696 L698 L691 L695 L644 | L651 L694 L693 L898 L894 L899 | L743 L933 L937 L669 L670 L653 | L660 L661 L659 L662 L657 L656 L655 L654 | L673 L729 L731 L728 L730 L674 L675 L671 | L677 L681 L687 L684 L683 L682 L679 L676 | L702 L721 L720 L718 L719 L706 L707 L704 | L744 L736 L738 L740 L742 L739 L737 L735 | L876 L873 L872 L931 L932 L741 | L745 L789 L790 L784 L870 L806 | L748 L822 L753 L752 L751 L750 L749 L747 | L756 L757 L759 L761 L763 L760 L758 L755 | L825 L823 L827 L830 L814 L764 | L765 L813 L817 L800 L773 L767 | L769 L801 L802 L841 L840 L938 L799 L770 | L772 L776 L781 L780 L779 L778 L774 L771 | L941 L943 L945 L947 L946 L775 | L783 L792 L796 L951 L953 L950 | L786 L791 L794 L795 L793 L785 | L803 L818 L821 L851 L852 L853 | L805 L807 L809 L871 L808 L828 L826 L804 | L810 L869 L868 L874 L875 L879 | L811 L812 L815 L833 L884 L819 L820 L816 | L867 L865 L885 L832 L831 L829 | L834 L942 L940 L939 L842 L836 | L846 L892 L893 L895 L839 L837 | L843 L845 L856 L860 L849 L848 L847 L844 | L886 L887 L888 L889 L857 L858 L854 L850 | L855 L859 L901 L902 L904 L861 | L926 L923 L925 L891 L864 L862 | L863 L866 L883 L882 L881 L878 L877 L880 | L924 L918 L914 L915 L916 L921 L922 L890 | L907 L913 L910 L912 L911 L909 L908 L906 | L927 L930 L929 L936 L935 L934 | L956 L960 L959 L958 L957 L954 | L1110 L1088 L1091 L981 L990 L972 | L1089 L1090 L1086 L1082 L1083 L1085 L984 L976 | L982 L1084 L1058 L1030 L1028 L997 | L1002 L988 L986 L987 L985 L983 | L1021 L1022 L1025 L1027 L1023 L1032 L1019 L991 | L992 L1008 L1037 L1035 L1000 L1024 | L1010 L1011 L1015 L1012 L1009 L995 | L996 L999 L1006 L1004 L1003 L1001 L998 L1026 | L1013 L1014 L1018 L1042 L1045 L1043 | L1033 L1041 L1040 L1039 L1036 L1034 | L1052 L1075 L1096 L1095 L1093 L1050 | L1057 L1059 L1060 L1062 L1064 L1068 L1067 L1061 | L1063 L1092 L1087 L1105 L1071 L1065 | L1073 L1074 L1076 L1080 L1079 L1078 L1077 L1072 | L1102 L1103 L1104 L1106 L1109 L1108 L1107 L1101
equation "\"d13\" = d11"
equation "\"d14\" = d12"
equation "\"d42\" = d39"
equation "\"d44\" = d41"
equation "\"d62\" = d57"
equation "\"d65\" = d62"
equation "\"d68\" = d65"
equation "\"d104\" = d61"
equation "\"d87\" = d62"
equation "\"d109\" = d100"
equation "\"d26\" = d24"
equation "\"d28\" = d26"
equation "\"d91\" = d90"
equation "\"d97\" = d96"
equation "\"d99\" = d95"
equation "\"d100\" = d99"
equation "\"d24\" = 44.7"
equation "\"d96\" = 52.5"
equation "\"d95\" = 7.5"
body "Solid1"
